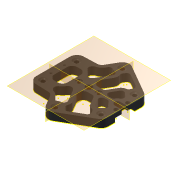
# Autodesk Inventor part: Part38
Saved by Autodesk Inventor 2016 (Build 200138000, 138)
## iProperties
Created: 2015-10-12
Part Number: Part38
Material: Nylon 6/6
Document SubType Name: Modeling
Designer: admin
Density: 1.13 g/cm^3
Appearance: Dark Gray
Mass: 19.0211 g
Surface Area: 121.419 cm^2
Volume: 16.8328 cm^3
Author: admin
Autodesk Inventor part; units mm, degrees
(part 1 of 2)
ref_plane "YZ Plane" through (0, 0, 0) normal (1, 0, 0) x (0, 1, 0)
ref_plane "XZ Plane" through (0, 0, 0) normal (0, 1, 0) x (-1, 0, 0)
ref_plane "XY Plane" through (0, 0, 0) normal (0, 0, 1) x (1, 0, 0)
sketch "Sketch1" plane through (0, 0, 0) normal (0, 0, 1) x (1, 0, 0)
  circle A0 centre (0, -12.97) radius 7.5 projected
  circle A1 centre (0, 21.03) radius 5
  circle A2 centre (-29.4449, 4.03) radius 5
  circle A3 centre (-29.4449, -29.97) radius 5
  circle A4 centre (0, -46.97) radius 5
  circle A5 centre (29.4449, -29.97) radius 5
  circle A6 centre (29.4449, 4.03) radius 5
  line L0 (3.5, 27.0921) -> (32.9449, 10.0921)
  line L1 (36.4449, 4.03) -> (36.4449, -29.97)
  line L2 (32.9449, -36.0322) -> (3.5, -53.0322)
  line L3 (-3.5, -53.0322) -> (-32.9449, -36.0322)
  line L4 (-36.4449, -29.97) -> (-36.4449, 4.03)
  line L5 (-32.9449, 10.0921) -> (-3.5, 27.0921)
  arc A7 (3.5, 27.0921) -> (-3.5, 27.0921) centre (0, 21.03) ccw
  arc A8 (-32.9449, 10.0921) -> (-36.4449, 4.03) centre (-29.4449, 4.03) ccw
  arc A9 (-36.4449, -29.97) -> (-32.9449, -36.0322) centre (-29.4449, -29.97) ccw
  arc A10 (-3.5, -53.0322) -> (3.5, -53.0322) centre (0, -46.97) ccw
  arc A11 (32.9449, -36.0322) -> (36.4449, -29.97) centre (29.4449, -29.97) ccw
  arc A12 (36.4449, 4.03) -> (32.9449, 10.0921) centre (29.4449, 4.03) ccw
  line L6 (-29.4449, 4.03) -> (0, 21.03)
  line L7 (0, 21.03) -> (29.4449, 4.03)
  line L8 (29.4449, 4.03) -> (29.4449, -29.97)
  line L9 (29.4449, -29.97) -> (0, -46.97)
  line L10 (0, -46.97) -> (-29.4449, -29.97)
  line L11 (-29.4449, -29.97) -> (-29.4449, 4.03)
  point P0 (0, 0)
  point P1 (36.4449, 8.0714)
  point P2 (36.4449, -34.0115)
  point P3 (0, -55.053)
  point P4 (-36.4449, -34.0115)
  point P5 (-36.4449, 8.0714)
  dimension "d1" = 10
  dimension "d2" = 10
  dimension "d3" = 10
  dimension "d4" = 10
  dimension "d5" = 10
  dimension "d6" = 10
  dimension "d55" = 2
  dimension "d56" = 2
  dimension "d57" = 2
  dimension "d58" = 2
  dimension "d59" = 2
  dimension "d60" = 2
  dimension "d61" = 34
  constraints: 24 end point, 12 centre point, 12 point on circle, 12 tangent, 10 point on line, 8 coincident, 5 equal radius, 13 other
  measures "d1" diameter of A1
  measures "d2" diameter of A2
  measures "d3" diameter of A3
  measures "d4" diameter of A4
  measures "d5" diameter of A5
  measures "d6" diameter of A6
  measures "d55" radial gap between concentric circles of A9 A3
  measures "d56" radial gap between concentric circles of A8 A2
  measures "d57" radial gap between concentric circles of A12 A6
  measures "d58" radial gap between concentric circles of A7 A1
  measures "d59" radial gap between concentric circles of A11 A5
  measures "d60" radial gap between concentric circles of A10 A4
  measures "d61" distance of L9.end L10.end
extrude "Extrusion1" add sketch "Sketch1" along normal blind 8 contours A0 | A1 L7 A6 L8 A5 L9 A4 L10 A3 L11 A2 L6 | L0 A12 L1 A11 L2 A10 L3 A9 L4 A8 L5 A7
sketch "Sketch2" plane through (0, 0, 8) normal (0, 0, 1) x (1, 0, 0)
  circle A0 centre (0, -12.97) radius 7.5 projected
  circle A1 centre (0, -12.97) radius 3.25
  point P0 (0, 0)
  dimension "d14" = 6.5
  constraints: 1 centre point, 1 coincident
  measures "d14" diameter of A1
extrude "Extrusion2" cut sketch "Sketch2" against normal blind 8 contours A1
sketch "Sketch4" plane through (0, 0, 8) normal (0, 0, 1) x (1, 0, 0)
  circle A0 centre (29.4449, 4.03) radius 5 projected
  circle A1 centre (29.4449, -29.97) radius 5 projected
  circle A2 centre (0, -46.97) radius 5 projected
  circle A3 centre (-29.4449, -29.97) radius 5 projected
  circle A4 centre (-29.4449, 4.03) radius 5 projected
  circle A5 centre (0, 21.03) radius 5 projected
  arc A6 (-32.9449, 10.0921) -> (-36.4449, 4.03) centre (-29.4449, 4.03) ccw projected
  arc A7 (-36.4449, -29.97) -> (-32.9449, -36.0322) centre (-29.4449, -29.97) ccw projected
  arc A8 (-3.5, -53.0322) -> (3.5, -53.0322) centre (0, -46.97) ccw projected
  arc A9 (32.9449, -36.0322) -> (36.4449, -29.97) centre (29.4449, -29.97) ccw projected
  arc A10 (36.4449, 4.03) -> (32.9449, 10.0921) centre (29.4449, 4.03) ccw projected
  arc A11 (3.5, 27.0921) -> (-3.5, 27.0921) centre (0, 21.03) ccw projected
  circle A12 centre (0, 21.03) radius 2
  circle A13 centre (29.4449, 4.03) radius 2
  circle A14 centre (-29.4449, 4.03) radius 2
  circle A15 centre (-29.4449, -29.97) radius 2
  circle A16 centre (0, -46.97) radius 2
  circle A17 centre (29.4449, -29.97) radius 2
  point P0 (0, 0)
  dimension "d19" = 4
  dimension "d20" = 4
  dimension "d21" = 4
  dimension "d22" = 4
  dimension "d23" = 4
  dimension "d24" = 4
  constraints: 6 centre point, 6 coincident
  measures "d19" diameter of A12
  measures "d20" diameter of A13
  measures "d21" diameter of A14
  measures "d22" diameter of A15
  measures "d23" diameter of A16
  measures "d24" diameter of A17
extrude "Extrusion4" add sketch "Sketch4" against normal blind 1.5
chamfer "Chamfer1" distance 2.2 angle 70 1 edges at (-3.25, -12.97, 0) measured on face at (-3.75, -12.97, 0)
ref_plane "Work Plane2" through (0, 28.03, 8) normal (1, 0, 0) x (0, -1, 0)
sketch "Sketch14" plane through (0, 0, 0) normal (0, 0, -1) x (-1, 0, 0)
  circle A0 centre (0, -12.97) radius 5.45 projected
  circle A1 centre (0, -12.97) radius 4.1
  point P0 (0, 0)
  dimension "d64" = 8.2
  constraints: 1 centre point, 1 coincident
  measures "d64" diameter of A1
extrude "Extrusion10" add sketch "Sketch14" against normal blind 5
ref_plane "Work Plane8" through (-36.4449, -12.97, 8) normal (0, -1, 0) x (0, 0, -1)
sketch "Sketch21" plane through (0, 0, 8) normal (0, 0, 1) x (1, 0, 0)
  circle A0 centre (-10, -12.97) radius 1.5
  circle A1 centre (10, -12.97) radius 1.5
  point P0 (0, 0)
  constraints: 2 centre point, 4 other
extrude "Extrusion17" cut sketch "Sketch21" against normal blind 8
sketch "Sketch26" plane through (0, 0, 8) normal (0, 0, 1) x (1, 0, 0)
  line L0 (36.4449, -29.97) -> (36.4449, 4.03) projected
  line L1 (43.9449, -12.97) -> (28.9449, -12.97) construction
  line L2 (43.9449, -9.97) -> (28.9449, -9.97)
  line L3 (28.9449, -15.97) -> (43.9449, -15.97)
  arc A0 (43.9449, -15.97) -> (43.9449, -9.97) centre (43.9449, -12.97) ccw
  arc A1 (28.9449, -9.97) -> (28.9449, -15.97) centre (28.9449, -12.97) ccw
  point P0 (0, 0)
  point P1 (36.4449, -12.97)
  dimension "d133" = 6
  dimension "d134" = 7.5
  constraints: 8 end point, 4 point on circle, 4 tangent, 2 centre point, 2 midpoint, 1 parallel, 1 perpendicular
  measures "d133" diameter of A1
  measures "d134" distance of L1.end point (36.445, -12.97)
extrude "Extrusion21" cut sketch "Sketch26" against normal blind 8
sketch "Sketch34" plane through (0, 0, 0) normal (0, 0, -1) x (-1, 0, 0)
  circle A0 centre (-33.4449, -6.97) radius 1.5
  circle A1 centre (-33.4449, -18.97) radius 1.5
  circle A2 centre (-33.4449, -6.97) radius 2
  circle A3 centre (-33.4449, -18.97) radius 2
  point P0 (0, 0)
  dimension "d175" = 4
  dimension "d176" = 4
  constraints: 4 centre point, 2 coincident, 4 other
  measures "d175" diameter of A2
  measures "d176" diameter of A3
extrude "Extrusion27" cut sketch "Sketch34" against normal blind 10 contours A0 | A1 | A2 | A3
sketch "Sketch35" plane through (0, 0, 0) normal (0, 0, -1) x (-1, 0, 0)
  circle A0 centre (-33.4449, -6.97) radius 2 projected
  circle A1 centre (-33.4449, -18.97) radius 2 projected
  line L0 (-36.4449, -9.97) -> (-36.4449, 4.03) projected
  line L1 (-36.4449, -29.97) -> (-36.4449, -15.97) projected
  line L2 (-29.4449, -6.97) -> (-29.4449, -18.97)
  arc A2 (-29.4449, -6.97) -> (-33.4449, -2.97) centre (-33.4449, -6.97) ccw
  arc A3 (-33.4449, -22.97) -> (-29.4449, -18.97) centre (-33.4449, -18.97) ccw
  line L3 (-36.4449, -2.97) -> (-33.4449, -2.97)
  line L4 (-36.4449, -22.97) -> (-33.4449, -22.97)
  line L5 (-36.4449, -2.97) -> (-36.4449, -22.97)
  point P0 (0, 0)
  constraints: 8 end point, 4 point on circle, 4 tangent, 2 centre point, 2 coincident, 2 midpoint, 1 collinear
extrude "Extrusion28" cut sketch "Sketch35" against normal blind 4
sketch "Sketch36" plane through (0, 0, 0) normal (0, 0, -1) x (-1, 0, 0)
  ellipse E0 centre (31.6453, -6.0284) end of major axis (31.6453, -7.5284) minor radius 1.4998 (31.6715, -7.5282) -> (31.6715, -4.5286) ccw
  ellipse E1 centre (31.6453, -19.9117) end of major axis (31.6453, -21.4117) minor radius 1.4998 (31.6715, -21.4115) -> (31.6715, -18.4119) ccw
  circle A0 centre (31.6453, -6.0284) radius 1.2
  circle A1 centre (31.6453, -19.9117) radius 1.2
  point P0 (0, 0)
  dimension "d183" = 2.4
  dimension "d184" = 2.4
  constraints: 2 centre point, 2 coincident, 14 other
  measures "d183" diameter of A0
  measures "d184" diameter of A1
extrude "Extrusion29" cut sketch "Sketch36" against normal blind 8
ref_plane "Work Plane10" through (0, 0, 11.5) normal (0, 0, 1) x (1, 0, 0)
sketch "Sketch38" plane through (0, 0, 11.5) normal (0, 0, 1) x (1, 0, 0)
  circle A0 centre (0, 21.03) radius 2 projected
  circle A1 centre (0, 21.03) radius 5
  line L0 (4.8928, 20) -> (-4.8928, 22.0599)
  point P0 (0, 0)
  dimension "d206" = 10
  constraints: 2 end point, 2 point on circle, 1 centre point, 1 coincident, 1 midpoint
  measures "d206" diameter of A1
revolve "Revolution2" cut sketch "Sketch38" angle 360 about axis through (4.8928, 20, 11.5) along (-0.978554, 0.2059906, 0) picked at (-0.0936, 21.69) picked at (-3.73, 22.3924) contours A0 L0 | A0 L0 A1
pattern_circular "Circular Pattern3" count 6 over 360 about axis through (0, -12.97, 8) along (0, 0, -1) of "Revolution2"
thread "Thread3" size "M3x0.5" class "6H" standard "ANSI Metric M Profile" full length
thread "Thread4" size "M3x0.5" class "6H" standard "ANSI Metric M Profile" full length
sketch "Sketch39" plane through (0, 0, 8) normal (0, 0, 1) x (1, 0, 0)
  circle A0 centre (10, -12.97) radius 1.5 projected
  circle A1 centre (-10, -12.97) radius 1.5 projected
  circle A2 centre (-10, -12.97) radius 3
  circle A3 centre (10, -12.97) radius 3
  point P0 (0, 0)
  dimension "d215" = 6
  dimension "d216" = 6
  constraints: 2 centre point, 2 coincident
  measures "d215" diameter of A2
  measures "d216" diameter of A3
extrude "Extrusion31" cut sketch "Sketch39" against normal blind 1
sketch "Sketch41" plane through (0, 0, 8) normal (0, 0, 1) x (1, 0, 0)
  line L0 (-3.5, 27.0921) -> (-32.9449, 10.0921) projected
  arc A0 (-32.9449, 10.0921) -> (-36.4449, 4.03) centre (-29.4449, 4.03) ccw projected
  line L1 (-36.4449, 4.03) -> (-36.4449, -29.97) projected
  arc A1 (-36.4449, -29.97) -> (-32.9449, -36.0322) centre (-29.4449, -29.97) ccw projected
  line L2 (-32.9449, -36.0322) -> (-3.5, -53.0322) projected
  ellipse E0 centre (-29.4445, 4.2702) end of major axis (-36.4456, 4.2702) minor radius 7 (-31.374, 10.9991) -> (-36.4456, 4.2702) ccw
  ellipse E1 centre (-29.4445, -30.2102) end of major axis (-22.4434, -30.2102) minor radius 7 (-36.4456, -30.2102) -> (-31.3743, -36.939) ccw
  line L3 (-36.4456, 4.2702) -> (-36.4456, -30.2102)
  point P0 (0, 0)
  constraints: 2 end point, 2 point on line, 2 vertical, 1 parallel, 14 other
extrude "Extrusion33" add sketch "Sketch41" against normal blind 8
sketch "Sketch42" plane through (0, 0, 8) normal (0, 0, 1) x (1, 0, 0)
  line L0 (28.9449, -9.97) -> (36.4449, -9.97) projected
  line L1 (32.9449, 10.0921) -> (3.5, 27.0921) projected
  arc A0 (3.5, 27.0921) -> (-3.5, 27.0921) centre (0, 21.03) ccw projected
  line L2 (-3.5, 27.0921) -> (-31.374, 10.9991) projected
  ellipse E0 centre (-29.4445, 4.2702) end of major axis (-36.4456, 4.2702) minor radius 7 (-31.374, 10.9991) -> (-36.4456, 4.2702) ccw projected
  ellipse E1 centre (-29.4445, -30.2102) end of major axis (-22.4434, -30.2102) minor radius 7 (-36.4456, -30.2102) -> (-31.3743, -36.939) ccw projected
  line L3 (-31.3743, -36.939) -> (-3.5, -53.0322) projected
  arc A1 (-3.5, -53.0322) -> (3.5, -53.0322) centre (0, -46.97) ccw projected
  line L4 (3.5, -53.0322) -> (32.9449, -36.0322) projected
  line L5 (36.4449, -15.97) -> (28.9449, -15.97) projected
  line L6 (-29.6889, 11.2659) -> (-16.1615, 11.7383)
  line L7 (-29.6889, -37.2059) -> (-16.1615, -37.6783)
  arc A2 (-31.3743, -36.939) -> (-29.6554, -37.2071) centre (-29.4445, -30.2102) ccw
  arc A3 (-29.6554, 11.2671) -> (-31.374, 10.9991) centre (-29.4445, 4.2702) ccw
  line L8 (-6.0622, -50.47) -> (-12.0059, -40.1753)
  line L9 (-6.0622, 24.53) -> (-12.0058, 14.2353)
  arc A4 (-3.5, 27.0921) -> (-6.0622, 24.53) centre (0, 21.03) ccw
  arc A5 (-6.0622, -50.47) -> (-3.5, -53.0322) centre (0, -46.97) ccw
  line L10 (-31.374, 10.9991) -> (-3.5, 27.0921)
  line L11 (-31.3743, -36.939) -> (-3.5, -53.0322)
  arc A6 (-12.0059, -40.1753) -> (-16.1615, -37.6783) centre (-16.336, -42.6753) ccw
  arc A7 (-16.1615, 11.7383) -> (-12.0058, 14.2353) centre (-16.336, 16.7353) ccw
  point P0 (0, 0)
  dimension "d234" = 2
  dimension "d235" = 2
  dimension "d236" = 60
  dimension "d237" = 60
  dimension "d238" = 5
  constraints: 15 end point, 14 point on circle, 10 tangent, 6 centre point, 4 coincident, 4 point on line, 2 collinear, 1 equal radius, 7 other
  measures "d234" angle of L0 L6
  measures "d235" angle of L7 L5
  measures "d236" angle of L0 L9
  measures "d237" angle of L8 L5
  measures "d238" radius of A6
extrude "Extrusion34" cut sketch "Sketch42" against normal blind 8
sketch "Sketch43" plane through (0, 0, 8) normal (0, 0, 1) x (1, 0, 0)
  arc A0 (28.9449, -9.97) -> (28.9449, -15.97) centre (28.9449, -12.97) ccw projected
  line L0 (28.9449, -9.97) -> (36.4449, -9.97) projected
  line L1 (-6.0622, 24.53) -> (-12.0058, 14.2353) projected
  arc A1 (-16.1615, 11.7383) -> (-12.0058, 14.2353) centre (-16.336, 16.7353) ccw projected
  arc A2 (-12.0059, -40.1753) -> (-16.1615, -37.6783) centre (-16.336, -42.6753) ccw projected
  circle A3 centre (10, -12.97) radius 3 projected
  circle A4 centre (0, 21.03) radius 3.5707 projected
  circle A5 centre (33.4449, -18.97) radius 2 projected
  circle A6 centre (0, -12.97) radius 3.25 projected
  line L2 (-23.6453, -1.2367) -> (-20, -1.2367)
  line L3 (-15, -6.2367) -> (-15, -19.7033)
  line L4 (-20, -24.7033) -> (-23.6453, -24.7033)
  line L5 (-28.6453, -19.7033) -> (-28.6453, -6.2367)
  arc A7 (-23.6453, -1.2367) -> (-28.6453, -6.2367) centre (-23.6453, -6.2367) ccw
  arc A8 (-15, -6.2367) -> (-20, -1.2367) centre (-20, -6.2367) ccw
  arc A9 (-20, -24.7033) -> (-15, -19.7033) centre (-20, -19.7033) ccw
  arc A10 (-28.6453, -19.7033) -> (-23.6453, -24.7033) centre (-23.6453, -19.7033) ccw
  line L6 (4.0415, -17.97) -> (8.6603, -17.97)
  line L7 (4.0415, -7.97) -> (8.6603, -7.97)
  line L8 (31.5084, -19.47) -> (32.9449, -19.47)
  arc A11 (-8.9748, -38.4253) -> (-14.507, -34.3744) centre (-16.336, -42.6753) ccw
  arc A12 (-14.507, 8.4344) -> (-8.9747, 12.4853) centre (-16.336, 16.7353) ccw
  line L9 (-22.7372, 2.2633) -> (-22.7383, 2.2633)
  arc A13 (-15.6795, -27.0233) -> (-12.4713, -23.6489) centre (-20, -19.7033) ccw
  arc A14 (-12.4713, -2.2911) -> (-15.6795, 1.0833) centre (-20, -6.2367) ccw
  line L10 (1.4796, -35.5328) -> (-5.4642, -23.5057)
  line L11 (1.4796, 9.5927) -> (-5.4642, -2.4343)
  arc A15 (-14.507, 8.4344) -> (-15.6795, 1.0833) centre (-13.6463, 4.5281) ccw
  arc A16 (-15.6795, -27.0233) -> (-14.507, -34.3744) centre (-13.6463, -30.4681) ccw
  arc A17 (-5.4642, -23.5057) -> (-12.4713, -23.6489) centre (-8.9283, -25.5057) ccw
  arc A18 (-12.4713, -2.2911) -> (-5.4642, -2.4343) centre (-8.9283, -0.4343) ccw
  line L12 (17.7535, -11.22) -> (20.7176, -11.22)
  line L13 (17.7535, -14.72) -> (20.7176, -14.72)
  arc A19 (25.8495, -7.2544) -> (23.3157, -9.72) centre (28.9449, -12.97) ccw
  arc A20 (23.3157, -16.22) -> (25.8495, -18.6857) centre (28.9449, -12.97) ccw
  arc A21 (25.8495, -7.2544) -> (25.9281, -2.0225) centre (24.4209, -4.6164) ccw
  arc A22 (25.9281, -23.9176) -> (25.8495, -18.6857) centre (24.4209, -21.3237) ccw
  line L14 (-23.5069, -33.9197) -> (-23.5081, -33.9196)
  line L15 (-0.2887, -25.47) -> (4.5273, -33.8116)
  line L16 (4.5273, 7.8715) -> (-0.2887, -0.47)
  arc A23 (1.4796, 9.5927) -> (-0.7829, 14.0739) centre (-1.1185, 11.0927) ccw
  arc A24 (-3.7987, 15.1504) -> (-8.0248, 14.1305) centre (-5.4268, 12.6305) ccw
  line L17 (-8.9747, 12.4853) -> (-8.0248, 14.1305)
  arc A25 (-3.7987, 15.1504) -> (-0.7829, 14.0739) centre (0, 21.03) ccw
  arc A26 (-8.0248, -40.0706) -> (-3.7987, -41.0905) centre (-5.4268, -38.5706) ccw
  arc A27 (-0.7829, -40.014) -> (1.4796, -35.5328) centre (-1.1185, -37.0328) ccw
  line L18 (-8.0248, -40.0706) -> (-8.9748, -38.4253)
  arc A28 (-0.7829, -40.014) -> (-3.7987, -41.0905) centre (0, -46.97) ccw
  arc A29 (-0.2887, -0.47) -> (4.0415, -7.97) centre (4.0415, -2.97) ccw
  arc A30 (4.0415, -17.97) -> (-0.2887, -25.47) centre (4.0415, -22.97) ccw
  line L19 (-12.0059, -40.1753) -> (-6.0622, -50.47) projected
  line L20 (18.8001, -0.4073) -> (15.1554, -6.72)
  line L21 (18.8001, -25.5328) -> (15.1554, -19.22)
  line L22 (15.93, 1.6215) -> (11.2583, -6.47)
  line L23 (11.2583, -19.47) -> (15.93, -27.5616)
  arc A31 (15.1554, -6.72) -> (17.7535, -11.22) centre (17.7535, -8.22) ccw
  arc A32 (17.7535, -14.72) -> (15.1554, -19.22) centre (17.7535, -17.72) ccw
  arc A33 (18.8001, -25.5328) -> (23.8122, -25.814) centre (21.3982, -24.0328) ccw
  arc A34 (23.8122, -0.1261) -> (18.8001, -0.4073) centre (21.3982, -1.9073) ccw
  arc A35 (20.7176, -11.22) -> (23.3157, -9.72) centre (20.7176, -8.22) ccw
  arc A36 (23.3157, -16.22) -> (20.7176, -14.72) centre (20.7176, -17.72) ccw
  arc A37 (23.8122, -0.1261) -> (25.9281, -2.0225) centre (29.4449, 4.03) ccw
  arc A38 (25.9281, -23.9176) -> (23.8122, -25.814) centre (29.4449, -29.97) ccw
  line L24 (13.4413, 17.311) -> (19.5035, 13.811)
  arc A39 (8.6603, -7.97) -> (11.2583, -6.47) centre (8.6603, -4.97) ccw
  arc A40 (11.2583, -19.47) -> (8.6603, -17.97) centre (8.6603, -20.97) ccw
  line L25 (13.4413, 17.311) -> (7, 21.03)
  line L26 (19.5035, 13.811) -> (25.9449, 10.0921)
  arc A41 (4.4941, 7.8139) -> (3.9036, 15.2194) centre (-1.1185, 11.0927) ccw
  arc A42 (22.4616, 4.5132) -> (15.6081, 1.0639) centre (21.3982, -1.9073) ccw
  arc A43 (25.9449, 10.0921) -> (22.4616, 4.5132) centre (29.4449, 4.03) ccw
  arc A44 (3.9036, 15.2194) -> (7, 21.03) centre (0, 21.03) ccw
  line L27 (0, -12.97) -> (10, -12.97)
  line L28 (13.4413, -43.2511) -> (7, -46.97)
  line L29 (19.5035, -39.7511) -> (25.9449, -36.0322)
  arc A45 (3.9036, -41.1595) -> (4.4941, -33.754) centre (-1.1185, -37.0328) ccw
  arc A46 (15.6081, -27.004) -> (22.4616, -30.4533) centre (21.3982, -24.0328) ccw
  arc A47 (22.4616, -30.4533) -> (25.9449, -36.0322) centre (29.4449, -29.97) ccw
  arc A48 (7, -46.97) -> (3.9036, -41.1595) centre (0, -46.97) ccw
  line L30 (13.4413, -43.2511) -> (19.5035, -39.7511)
  point P0 (0, -46.97)
  point P1 (29.4449, -29.97)
  point P2 (0, 21.03)
  point P3 (-29.4445, -30.2102)
  point P4 (0, 0)
  point P5 (10, -17.97)
  point P6 (10, -7.97)
  point P7 (22.6849, -11.22)
  point P8 (22.6849, -14.72)
  dimension "d243" = 5
  dimension "d248" = 3.5
  dimension "d249" = 8
  dimension "d250" = 8
  dimension "d251" = 8
  dimension "d253" = 8
  dimension "d254" = 3.5
  dimension "d255" = 1.75
  dimension "d256" = 6
  dimension "d261" = 3.5
  dimension "d262" = 3.5
  dimension "d263" = 6
  dimension "d264" = 6
  dimension "d265" = 6
  dimension "d266" = 6
  dimension "d267" = 10
  dimension "d268" = 10
  dimension "d269" = 17.5
  dimension "d270" = 17.5
  dimension "d271" = 3.5
  dimension "d272" = 3.5
  dimension "d273" = 6
  dimension "d274" = 6
  dimension "d275" = 6
  dimension "d276" = 6
  dimension "d277" = 3
  constraints: 90 point on circle, 57 end point, 42 centre point, 40 tangent, 10 symmetric about line, 8 parallel, 6 point on line, 5 coincident, 4 equal radius, 3 collinear, 2 perpendicular, 1 horizontal, 6 other
  measures "d243" radius of A7
  measures "d248" radial gap between concentric circles of A8 A14
  measures "d249" diameter of A15
  measures "d250" diameter of A16
  measures "d251" diameter of A17
  measures "d253" diameter of A18
  measures "d254" distance between parallel lines of L12 L13
  measures "d255" distance from line of L27.end L12
  measures "d256" diameter of A21
  measures "d261" distance between parallel lines of L10 L15
  measures "d262" distance between parallel lines of L11 L16
  measures "d263" diameter of A23
  measures "d264" diameter of A24
  measures "d265" diameter of A26
  measures "d266" diameter of A27
  measures "d267" diameter of A29
  measures "d268" diameter of A30
  measures "d269" distance between parallel lines of L19 L15
  measures "d270" distance between parallel lines of L1 L16
  measures "d271" distance between parallel lines of L20 L22
  measures "d272" distance between parallel lines of L21 L23
  measures "d273" diameter of A31
  measures "d274" diameter of A32
  measures "d275" diameter of A33
  measures "d276" diameter of A34
  measures "d277" radius of A35
extrude "Extrusion35" cut sketch "Sketch43" against normal blind 8 contours L2 A8 L3 A9 L4 A10 L5 A7 | L6 A40 L23 A46 A47 L29 L30 L28 A48 A45 L15 A30 | L23 A46 | A29 L16 A41 A44 L25 L24 L26 A43 A42 L22 A39 L7 | A11 A16 A13 A17 L10 A27 A28 A26 L18 | A12 L17 A24 A25 A23 L11 A18 A14 A15 | A31 L20 A34 A37 A21 A19 A35 L12 | L13 A36 A20 A22 A38 A33 L21 A32
fillet "Fillet8" radius 3 8 edges at (25.9449, 10.0921, 4) (22.4616, 4.5132, 4) (7, 21.03, 4) (3.9036, 15.2194, 4) (22.4616, -30.4533, 4) (25.9449, -36.0322, 4) (3.9036, -41.1595, 4) (7, -46.97, 4)
sketch "Sketch45" plane through (0, 0, 0) normal (0, 0, -1) x (-1, 0, 0)
  arc A0 (-11.2583, -6.47) -> (-8.6603, -7.97) centre (-8.6603, -4.97) ccw projected
  line L0 (-11.2583, -6.47) -> (-15.6081, 1.0639) projected
  arc A1 (-15.6081, 1.0639) -> (-20.4883, 4.5367) centre (-21.3982, -1.9073) ccw projected
  arc A2 (-22.8817, 6.4641) -> (-20.4883, 4.5367) centre (-20.0689, 7.5073) ccw projected
  arc A3 (-22.8817, 6.4641) -> (-23.5653, 7.8287) centre (-29.4449, 4.03) ccw projected
  arc A4 (-22.5454, 12.0548) -> (-23.5653, 7.8287) centre (-21.0454, 9.4567) ccw projected
  line L1 (-22.5454, 12.0548) -> (-10.3994, 19.0673) projected
  arc A5 (-6.2296, 17.8374) -> (-10.3994, 19.0673) centre (-8.8994, 16.4692) ccw projected
  arc A6 (-6.2296, 17.8374) -> (-5.3856, 16.5583) centre (0, 21.03) ccw projected
  arc A7 (-4.9109, 13.5211) -> (-5.3856, 16.5583) centre (-7.6937, 14.6419) ccw projected
  arc A8 (-4.9109, 13.5211) -> (-4.4941, 7.8139) centre (1.1185, 11.0927) ccw projected
  line L2 (-4.4941, 7.8139) -> (0.2887, -0.47) projected
  arc A9 (-4.0415, -7.97) -> (0.2887, -0.47) centre (-4.0415, -2.97) ccw projected
  line L3 (-4.0415, -7.97) -> (-8.6603, -7.97) projected
  line L4 (8.9748, -38.4253) -> (8.0248, -40.0706) projected
  arc A10 (3.7987, -41.0905) -> (8.0248, -40.0706) centre (5.4268, -38.5706) ccw projected
  arc A11 (3.7987, -41.0905) -> (0.7829, -40.014) centre (0, -46.97) ccw projected
  arc A12 (-1.4796, -35.5328) -> (0.7829, -40.014) centre (1.1185, -37.0328) ccw projected
  line L5 (-1.4796, -35.5328) -> (5.4642, -23.5057) projected
  arc A13 (12.4713, -23.6489) -> (5.4642, -23.5057) centre (8.9283, -25.5057) ccw projected
  arc A14 (12.4713, -23.6489) -> (15.6795, -27.0233) centre (20, -19.7033) ccw projected
  arc A15 (14.507, -34.3744) -> (15.6795, -27.0233) centre (13.6463, -30.4681) ccw projected
  arc A16 (14.507, -34.3744) -> (8.9748, -38.4253) centre (16.336, -42.6753) ccw projected
  arc A17 (-25.9281, -2.0225) -> (-23.8122, -0.1261) centre (-29.4449, 4.03) ccw projected
  arc A18 (-18.8001, -0.4073) -> (-23.8122, -0.1261) centre (-21.3982, -1.9073) ccw projected
  line L6 (-18.8001, -0.4073) -> (-15.1554, -6.72) projected
  arc A19 (-17.7535, -11.22) -> (-15.1554, -6.72) centre (-17.7535, -8.22) ccw projected
  line L7 (-17.7535, -11.22) -> (-20.7176, -11.22) projected
  arc A20 (-23.3157, -9.72) -> (-20.7176, -11.22) centre (-20.7176, -8.22) ccw projected
  arc A21 (-23.3157, -9.72) -> (-25.8495, -7.2544) centre (-28.9449, -12.97) ccw projected
  arc A22 (-25.9281, -2.0225) -> (-25.8495, -7.2544) centre (-24.4209, -4.6164) ccw projected
  arc A23 (-20.7176, -14.72) -> (-23.3157, -16.22) centre (-20.7176, -17.72) ccw projected
  line L8 (-20.7176, -14.72) -> (-17.7535, -14.72) projected
  arc A24 (-15.1554, -19.22) -> (-17.7535, -14.72) centre (-17.7535, -17.72) ccw projected
  line L9 (-15.1554, -19.22) -> (-18.8001, -25.5328) projected
  arc A25 (-23.8122, -25.814) -> (-18.8001, -25.5328) centre (-21.3982, -24.0328) ccw projected
  arc A26 (-23.8122, -25.814) -> (-25.9281, -23.9176) centre (-29.4449, -29.97) ccw projected
  arc A27 (-25.8495, -18.6857) -> (-25.9281, -23.9176) centre (-24.4209, -21.3237) ccw projected
  arc A28 (-25.8495, -18.6857) -> (-23.3157, -16.22) centre (-28.9449, -12.97) ccw projected
  arc A29 (15.6795, 1.0833) -> (14.507, 8.4344) centre (13.6463, 4.5281) ccw projected
  arc A30 (15.6795, 1.0833) -> (12.4713, -2.2911) centre (20, -6.2367) ccw projected
  arc A31 (5.4642, -2.4343) -> (12.4713, -2.2911) centre (8.9283, -0.4343) ccw projected
  line L10 (5.4642, -2.4343) -> (-1.4796, 9.5927) projected
  arc A32 (0.7829, 14.0739) -> (-1.4796, 9.5927) centre (1.1185, 11.0927) ccw projected
  arc A33 (0.7829, 14.0739) -> (3.7987, 15.1504) centre (0, 21.03) ccw projected
  arc A34 (8.0248, 14.1305) -> (3.7987, 15.1504) centre (5.4268, 12.6305) ccw projected
  line L11 (8.0248, 14.1305) -> (8.9747, 12.4853) projected
  arc A35 (8.9747, 12.4853) -> (14.507, 8.4344) centre (16.336, 16.7353) ccw projected
  arc A36 (23.6453, -24.7033) -> (28.6453, -19.7033) centre (23.6453, -19.7033) ccw projected
  line L12 (23.6453, -24.7033) -> (20, -24.7033) projected
  arc A37 (15, -19.7033) -> (20, -24.7033) centre (20, -19.7033) ccw projected
  line L13 (15, -19.7033) -> (15, -6.2367) projected
  arc A38 (20, -1.2367) -> (15, -6.2367) centre (20, -6.2367) ccw projected
  line L14 (20, -1.2367) -> (23.6453, -1.2367) projected
  arc A39 (28.6453, -6.2367) -> (23.6453, -1.2367) centre (23.6453, -6.2367) ccw projected
  line L15 (28.6453, -6.2367) -> (28.6453, -19.7033) projected
  arc A40 (0.2887, -25.47) -> (-4.0415, -17.97) centre (-4.0415, -22.97) ccw projected
  line L16 (0.2887, -25.47) -> (-4.5273, -33.8116) projected
  arc A41 (-4.5273, -33.8116) -> (-4.9109, -39.4612) centre (1.1185, -37.0328) ccw projected
  arc A42 (-5.3856, -42.4984) -> (-4.9109, -39.4612) centre (-7.6937, -40.582) ccw projected
  arc A43 (-5.3856, -42.4984) -> (-6.2296, -43.7775) centre (0, -46.97) ccw projected
  arc A44 (-10.3994, -45.0074) -> (-6.2296, -43.7775) centre (-8.8994, -42.4093) ccw projected
  line L17 (-10.3994, -45.0074) -> (-22.5454, -37.9949) projected
  arc A45 (-23.5653, -33.7688) -> (-22.5454, -37.9949) centre (-21.0454, -35.3968) ccw projected
  arc A46 (-23.5653, -33.7688) -> (-22.8817, -32.4042) centre (-29.4449, -29.97) ccw projected
  arc A47 (-20.4883, -30.4768) -> (-22.8817, -32.4042) centre (-20.0689, -33.4474) ccw projected
  arc A48 (-20.4883, -30.4768) -> (-15.93, -27.5616) centre (-21.3982, -24.0328) ccw projected
  line L18 (-15.93, -27.5616) -> (-11.2583, -19.47) projected
  arc A49 (-8.6603, -17.97) -> (-11.2583, -19.47) centre (-8.6603, -20.97) ccw projected
  line L19 (-8.6603, -17.97) -> (-4.0415, -17.97) projected
  circle A50 centre (-29.4449, 4.03) radius 5 projected
  circle A51 centre (-29.4449, -29.97) radius 5 projected
  circle A52 centre (0, -46.97) radius 5 projected
  circle A53 centre (29.4449, -29.97) radius 5 projected
  circle A54 centre (29.4449, 4.03) radius 5 projected
  circle A55 centre (0, 21.03) radius 5 projected
  circle A56 centre (0, -12.97) radius 4.1 projected
  circle A57 centre (-10, -12.97) radius 1.5 projected
  circle A58 centre (10, -12.97) radius 1.5 projected
  circle A59 centre (31.6453, -19.9117) radius 1.2 projected
  circle A60 centre (31.6453, -6.0284) radius 1.2 projected
  arc A61 (-3.5, -53.0322) -> (6.0622, -50.47) centre (0, -46.97) ccw projected
  line L20 (6.0622, -50.47) -> (12.0059, -40.1753) projected
  arc A62 (16.1615, -37.6783) -> (12.0059, -40.1753) centre (16.336, -42.6753) ccw projected
  line L21 (16.1615, -37.6783) -> (29.6554, -37.2071) projected
  arc A63 (29.6554, -37.2071) -> (31.3743, -36.939) centre (29.4445, -30.2102) ccw projected
  ellipse E0 centre (29.4445, -30.2102) end of major axis (22.4434, -30.2102) minor radius 7 (31.3743, -36.939) -> (36.4456, -30.2102) ccw projected
  line L22 (36.4456, -30.2102) -> (36.4456, 4.2702) projected
  ellipse E1 centre (29.4445, 4.2702) end of major axis (36.4456, 4.2702) minor radius 7 (36.4456, 4.2702) -> (31.374, 10.9991) ccw projected
  arc A64 (31.374, 10.9991) -> (29.6554, 11.2671) centre (29.4445, 4.2702) ccw projected
  line L23 (29.6554, 11.2671) -> (16.1615, 11.7383) projected
  arc A65 (12.0058, 14.2353) -> (16.1615, 11.7383) centre (16.336, 16.7353) ccw projected
  line L24 (12.0058, 14.2353) -> (6.0622, 24.53) projected
  arc A66 (6.0622, 24.53) -> (-3.5, 27.0921) centre (0, 21.03) ccw projected
  line L25 (-32.9449, 10.0921) -> (-3.5, 27.0921) projected
  arc A67 (-32.9449, 10.0921) -> (-36.4449, 4.03) centre (-29.4449, 4.03) ccw projected
  line L26 (-36.4449, -2.97) -> (-36.4449, 4.03) projected
  line L27 (-36.4449, -2.97) -> (-33.4449, -2.97) projected
  arc A68 (-29.4449, -6.97) -> (-33.4449, -2.97) centre (-33.4449, -6.97) ccw projected
  line L28 (-29.4449, -6.97) -> (-29.4449, -9.97) projected
  line L29 (-29.4449, -9.97) -> (-28.9449, -9.97) projected
  arc A69 (-28.9449, -15.97) -> (-28.9449, -9.97) centre (-28.9449, -12.97) ccw projected
  line L30 (-28.9449, -15.97) -> (-29.4449, -15.97) projected
  line L31 (-29.4449, -15.97) -> (-29.4449, -18.97) projected
  arc A70 (-33.4449, -22.97) -> (-29.4449, -18.97) centre (-33.4449, -18.97) ccw projected
  line L32 (-33.4449, -22.97) -> (-36.4449, -22.97) projected
  line L33 (-36.4449, -29.97) -> (-36.4449, -22.97) projected
  arc A71 (-36.4449, -29.97) -> (-32.9449, -36.0322) centre (-29.4449, -29.97) ccw projected
  line L34 (-3.5, -53.0322) -> (-32.9449, -36.0322) projected
  circle A72 centre (0.9, -50.57) radius 1.5
  circle A73 centre (-0.9, -50.57) radius 1.5
  point P0 (0, 0)
  dimension "d282" = 3
  dimension "d283" = 3
  dimension "d284" = 0.9
  dimension "d285" = 0.9
  dimension "d286" = 3.6
  dimension "d287" = 3.6
  constraints: 2 centre point, 2 other
  measures "d282" diameter of A72
  measures "d283" diameter of A73
  measures "d284" horizontal distance of A11.centre A72.centre
  measures "d285" horizontal distance of A11.centre A73.centre
  measures "d286" vertical distance of A72.centre A11.centre
  measures "d287" vertical distance of A11.centre A73.centre
extrude "Extrusion36" cut sketch "Sketch45" against normal up to surface (6.5 mm away) contours A73 A72 A52 | A52 A73 | A72 A52 | A52 A72 A73 | A73 A72 picked at (-1.4361, -51.2929) picked at (1.4337, -51.2979)
sketch "Sketch46" plane through (0, 0, 0) normal (0, 0, -1) x (-1, 0, 0)
  arc A0 (-3.5, -53.0322) -> (6.0622, -50.47) centre (0, -46.97) ccw projected
  line L0 (6.0622, -50.47) -> (12.0059, -40.1753) projected
  arc A1 (16.1615, -37.6783) -> (12.0059, -40.1753) centre (16.336, -42.6753) ccw projected
  line L1 (16.1615, -37.6783) -> (29.6554, -37.2071) projected
  arc A2 (29.6554, -37.2071) -> (31.3743, -36.939) centre (29.4445, -30.2102) ccw projected
  ellipse E0 centre (29.4445, -30.2102) end of major axis (22.4434, -30.2102) minor radius 7 (31.3743, -36.939) -> (36.4456, -30.2102) ccw projected
  line L2 (36.4456, -30.2102) -> (36.4456, 4.2702) projected
  ellipse E1 centre (29.4445, 4.2702) end of major axis (36.4456, 4.2702) minor radius 7 (36.4456, 4.2702) -> (31.374, 10.9991) ccw projected
  arc A3 (31.374, 10.9991) -> (29.6554, 11.2671) centre (29.4445, 4.2702) ccw projected
  line L3 (29.6554, 11.2671) -> (16.1615, 11.7383) projected
  arc A4 (12.0058, 14.2353) -> (16.1615, 11.7383) centre (16.336, 16.7353) ccw projected
  line L4 (12.0058, 14.2353) -> (6.0622, 24.53) projected
  arc A5 (6.0622, 24.53) -> (-3.5, 27.0921) centre (0, 21.03) ccw projected
  line L5 (-32.9449, 10.0921) -> (-3.5, 27.0921) projected
  arc A6 (-32.9449, 10.0921) -> (-36.4449, 4.03) centre (-29.4449, 4.03) ccw projected
  line L6 (-36.4449, -2.97) -> (-36.4449, 4.03) projected
  line L7 (-36.4449, -2.97) -> (-33.4449, -2.97) projected
  arc A7 (-29.4449, -6.97) -> (-33.4449, -2.97) centre (-33.4449, -6.97) ccw projected
  line L8 (-29.4449, -6.97) -> (-29.4449, -9.97) projected
  line L9 (-29.4449, -9.97) -> (-28.9449, -9.97) projected
  arc A8 (-28.9449, -15.97) -> (-28.9449, -9.97) centre (-28.9449, -12.97) ccw projected
  line L10 (-28.9449, -15.97) -> (-29.4449, -15.97) projected
  line L11 (-29.4449, -15.97) -> (-29.4449, -18.97) projected
  arc A9 (-33.4449, -22.97) -> (-29.4449, -18.97) centre (-33.4449, -18.97) ccw projected
  line L12 (-33.4449, -22.97) -> (-36.4449, -22.97) projected
  line L13 (-36.4449, -29.97) -> (-36.4449, -22.97) projected
  arc A10 (-36.4449, -29.97) -> (-32.9449, -36.0322) centre (-29.4449, -29.97) ccw projected
  line L14 (-3.5, -53.0322) -> (-32.9449, -36.0322) projected
  circle A11 centre (31.6453, -6.0284) radius 1.2 projected
  circle A12 centre (31.6453, -19.9117) radius 1.2 projected
  circle A13 centre (10, -12.97) radius 1.5 projected
  circle A14 centre (-10, -12.97) radius 1.5 projected
  circle A15 centre (0, -12.97) radius 4.1 projected
  circle A16 centre (0, 21.03) radius 5 projected
  circle A17 centre (29.4449, 4.03) radius 5 projected
  circle A18 centre (29.4449, -29.97) radius 5 projected
  circle A19 centre (-29.4449, -29.97) radius 5 projected
  circle A20 centre (-29.4449, 4.03) radius 5 projected
  arc A21 (0.2887, -25.47) -> (-4.0415, -17.97) centre (-4.0415, -22.97) ccw projected
  line L15 (0.2887, -25.47) -> (-4.5273, -33.8116) projected
  arc A22 (-4.5273, -33.8116) -> (-4.9109, -39.4612) centre (1.1185, -37.0328) ccw projected
  arc A23 (-5.3856, -42.4984) -> (-4.9109, -39.4612) centre (-7.6937, -40.582) ccw projected
  arc A24 (-5.3856, -42.4984) -> (-6.2296, -43.7775) centre (0, -46.97) ccw projected
  arc A25 (-10.3994, -45.0074) -> (-6.2296, -43.7775) centre (-8.8994, -42.4093) ccw projected
  line L16 (-10.3994, -45.0074) -> (-22.5454, -37.9949) projected
  arc A26 (-23.5653, -33.7688) -> (-22.5454, -37.9949) centre (-21.0454, -35.3968) ccw projected
  arc A27 (-23.5653, -33.7688) -> (-22.8817, -32.4042) centre (-29.4449, -29.97) ccw projected
  arc A28 (-20.4883, -30.4768) -> (-22.8817, -32.4042) centre (-20.0689, -33.4474) ccw projected
  arc A29 (-20.4883, -30.4768) -> (-15.93, -27.5616) centre (-21.3982, -24.0328) ccw projected
  line L17 (-15.93, -27.5616) -> (-11.2583, -19.47) projected
  arc A30 (-8.6603, -17.97) -> (-11.2583, -19.47) centre (-8.6603, -20.97) ccw projected
  line L18 (-8.6603, -17.97) -> (-4.0415, -17.97) projected
  arc A31 (23.6453, -24.7033) -> (28.6453, -19.7033) centre (23.6453, -19.7033) ccw projected
  line L19 (23.6453, -24.7033) -> (20, -24.7033) projected
  arc A32 (15, -19.7033) -> (20, -24.7033) centre (20, -19.7033) ccw projected
  line L20 (15, -19.7033) -> (15, -6.2367) projected
  arc A33 (20, -1.2367) -> (15, -6.2367) centre (20, -6.2367) ccw projected
  line L21 (20, -1.2367) -> (23.6453, -1.2367) projected
  arc A34 (28.6453, -6.2367) -> (23.6453, -1.2367) centre (23.6453, -6.2367) ccw projected
  line L22 (28.6453, -6.2367) -> (28.6453, -19.7033) projected
  arc A35 (15.6795, 1.0833) -> (14.507, 8.4344) centre (13.6463, 4.5281) ccw projected
  arc A36 (15.6795, 1.0833) -> (12.4713, -2.2911) centre (20, -6.2367) ccw projected
  arc A37 (5.4642, -2.4343) -> (12.4713, -2.2911) centre (8.9283, -0.4343) ccw projected
  line L23 (5.4642, -2.4343) -> (-1.4796, 9.5927) projected
  arc A38 (0.7829, 14.0739) -> (-1.4796, 9.5927) centre (1.1185, 11.0927) ccw projected
  arc A39 (0.7829, 14.0739) -> (3.7987, 15.1504) centre (0, 21.03) ccw projected
  arc A40 (8.0248, 14.1305) -> (3.7987, 15.1504) centre (5.4268, 12.6305) ccw projected
  line L24 (8.0248, 14.1305) -> (8.9747, 12.4853) projected
  arc A41 (8.9747, 12.4853) -> (14.507, 8.4344) centre (16.336, 16.7353) ccw projected
  arc A42 (-20.7176, -14.72) -> (-23.3157, -16.22) centre (-20.7176, -17.72) ccw projected
  line L25 (-20.7176, -14.72) -> (-17.7535, -14.72) projected
  arc A43 (-15.1554, -19.22) -> (-17.7535, -14.72) centre (-17.7535, -17.72) ccw projected
  line L26 (-15.1554, -19.22) -> (-18.8001, -25.5328) projected
  arc A44 (-23.8122, -25.814) -> (-18.8001, -25.5328) centre (-21.3982, -24.0328) ccw projected
  arc A45 (-23.8122, -25.814) -> (-25.9281, -23.9176) centre (-29.4449, -29.97) ccw projected
  arc A46 (-25.8495, -18.6857) -> (-25.9281, -23.9176) centre (-24.4209, -21.3237) ccw projected
  arc A47 (-25.8495, -18.6857) -> (-23.3157, -16.22) centre (-28.9449, -12.97) ccw projected
  arc A48 (-25.9281, -2.0225) -> (-23.8122, -0.1261) centre (-29.4449, 4.03) ccw projected
  arc A49 (-18.8001, -0.4073) -> (-23.8122, -0.1261) centre (-21.3982, -1.9073) ccw projected
  line L27 (-18.8001, -0.4073) -> (-15.1554, -6.72) projected
  arc A50 (-17.7535, -11.22) -> (-15.1554, -6.72) centre (-17.7535, -8.22) ccw projected
  line L28 (-17.7535, -11.22) -> (-20.7176, -11.22) projected
  arc A51 (-23.3157, -9.72) -> (-20.7176, -11.22) centre (-20.7176, -8.22) ccw projected
  arc A52 (-23.3157, -9.72) -> (-25.8495, -7.2544) centre (-28.9449, -12.97) ccw projected
  arc A53 (-25.9281, -2.0225) -> (-25.8495, -7.2544) centre (-24.4209, -4.6164) ccw projected
  line L29 (8.9748, -38.4253) -> (8.0248, -40.0706) projected
  arc A54 (3.7987, -41.0905) -> (8.0248, -40.0706) centre (5.4268, -38.5706) ccw projected
  arc A55 (3.7987, -41.0905) -> (0.7829, -40.014) centre (0, -46.97) ccw projected
  arc A56 (-1.4796, -35.5328) -> (0.7829, -40.014) centre (1.1185, -37.0328) ccw projected
  line L30 (-1.4796, -35.5328) -> (5.4642, -23.5057) projected
  arc A57 (12.4713, -23.6489) -> (5.4642, -23.5057) centre (8.9283, -25.5057) ccw projected
  arc A58 (12.4713, -23.6489) -> (15.6795, -27.0233) centre (20, -19.7033) ccw projected
  arc A59 (14.507, -34.3744) -> (15.6795, -27.0233) centre (13.6463, -30.4681) ccw projected
  arc A60 (14.507, -34.3744) -> (8.9748, -38.4253) centre (16.336, -42.6753) ccw projected
  arc A61 (-11.2583, -6.47) -> (-8.6603, -7.97) centre (-8.6603, -4.97) ccw projected
  line L31 (-11.2583, -6.47) -> (-15.6081, 1.0639) projected
  arc A62 (-15.6081, 1.0639) -> (-20.4883, 4.5367) centre (-21.3982, -1.9073) ccw projected
  arc A63 (-22.8817, 6.4641) -> (-20.4883, 4.5367) centre (-20.0689, 7.5073) ccw projected
  arc A64 (-22.8817, 6.4641) -> (-23.5653, 7.8287) centre (-29.4449, 4.03) ccw projected
  arc A65 (-22.5454, 12.0548) -> (-23.5653, 7.8287) centre (-21.0454, 9.4567) ccw projected
  line L32 (-22.5454, 12.0548) -> (-10.3994, 19.0673) projected
  arc A66 (-6.2296, 17.8374) -> (-10.3994, 19.0673) centre (-8.8994, 16.4692) ccw projected
  arc A67 (-6.2296, 17.8374) -> (-5.3856, 16.5583) centre (0, 21.03) ccw projected
  arc A68 (-4.9109, 13.5211) -> (-5.3856, 16.5583) centre (-7.6937, 14.6419) ccw projected
  arc A69 (-4.9109, 13.5211) -> (-4.4941, 7.8139) centre (1.1185, 11.0927) ccw projected
  line L33 (-4.4941, 7.8139) -> (0.2887, -0.47) projected
  arc A70 (-4.0415, -7.97) -> (0.2887, -0.47) centre (-4.0415, -2.97) ccw projected
  line L34 (-4.0415, -7.97) -> (-8.6603, -7.97) projected
  arc A71 (-2.0535, -51.5289) -> (-0.3334, -51.9589) centre (-0.9, -50.57) ccw projected
  arc A72 (2.0535, -51.5289) -> (-2.0535, -51.5289) centre (0, -46.97) ccw projected
  arc A73 (0.3334, -51.9589) -> (2.0535, -51.5289) centre (0.9, -50.57) ccw projected
  arc A74 (-0.3334, -51.9589) -> (0.3334, -51.9589) centre (0, -46.97) ccw projected
  arc A75 (0.029, -51.7913) -> (0.3334, -51.9589) centre (0.9, -50.57) ccw
  arc A76 (-0.3334, -51.9589) -> (-0.029, -51.7913) centre (-0.9, -50.57) ccw
  arc A77 (0.029, -51.7913) -> (-0.029, -51.7913) centre (0, -51.832) ccw
  point P0 (0, 0)
  dimension "d298" = 0.05
  constraints: 6 point on circle, 3 centre point, 2 coincident, 2 tangent, 2 other
  measures "d298" radius of A77
extrude "Extrusion37" add sketch "Sketch46" against normal up to surface (6.5 mm away) contours A76 A77 A75 A74
pattern_circular "Circular Pattern6" count 3 over 360 about axis through (0, -46.97, 8) along (0, 0, -1) of "Extrusion36", "Extrusion37"
pattern_circular "Circular Pattern7" count 6 over 360 about axis through (0, -12.97, 3.0222) along (0, 0, -1) of "Extrusion36", "Extrusion37", "Circular Pattern6"